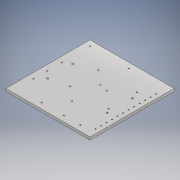
# Autodesk Inventor part: Base plate
Saved by Autodesk Inventor 2017 (Build 210142000, 142)
## iProperties
Created: 2016-09-16
Part Number: Base plate
Material: Aluminum 6061-AHC
Document SubType Name: Modeling
Designer: Andreas Fröderberg
Density: 2.7 g/cm^3
Appearance: Aluminum - Dark
Author: Andreas Fröderberg
Autodesk Inventor part; units mm, degrees
ref_plane "YZ Plane" through (0, 0, 0) normal (1, 0, 0) x (0, 1, 0)
ref_plane "XZ Plane" through (0, 0, 0) normal (0, 1, 0) x (-1, 0, 0)
ref_plane "XY Plane" through (0, 0, 0) normal (0, 0, 1) x (1, 0, 0)
sketch "Sketch1" plane through (0, 0, 0) normal (0, 0, 1) x (1, 0, 0)
  line L0 (0, 0) -> (305, 0)
  line L1 (305, 0) -> (305, 305)
  line L2 (305, 305) -> (0, 305)
  line L3 (0, 305) -> (0, 0)
  dimension "d0" = 305
  dimension "d1" = 305
  constraints: 8 end point, 2 parallel, 1 horizontal, 1 perpendicular
  measures "d0" distance of L2.end L1.end
  measures "d1" distance of L1.end L0.end
extrude "Extrusion1" add sketch "Sketch1" against normal blind 10
sketch "Sketch2" plane through (0, 0, 0) normal (0, 0, 1) x (1, 0, 0)
  line L0 (0, 305) -> (305, 305) projected
  line L1 (0, 305) -> (0, 0) projected
  point P0 (20, 285)
  point P1 (110, 225)
  dimension "d4" = 90
  dimension "d5" = 60
  dimension "d6" = 20
  dimension "d7" = 20
  measures "d4" horizontal distance of point (110, 225) point (20, 285)
  measures "d5" vertical distance of point (110, 225) point (20, 285)
  measures "d6" distance from line of L0 point (20, 285)
  measures "d7" distance from line of L1 point (20, 285)
hole "80x50" at (20, 285, 0) at (110, 225, 0) direction (0, 0, -1) diameter 4.134 depth 14.2 tip angle 118 thread size "M5x0.8" class "6H" standard "ISO Metric profile"
pattern_linear "Rectangular Pattern1" count 3 spacing 102.5 along (0, -1, 0) count 2 spacing 140 along (1, 0, 0) of "80x50"
sketch "Sketch4" plane through (0, 0, 0) normal (0, 0, 1) x (1, 0, 0)
  line L0 (0, 305) -> (0, 0) projected
  line L1 (305, 305) -> (0, 305) projected
  point P0 (290, 255)
  dimension "d40" = 290
  dimension "d41" = 50
  measures "d40" distance from line of L0 point (290, 255)
  measures "d41" distance from line of L1 point (290, 255)
hole "Magasin" at (290, 255, 0) direction (0, 0, -1) diameter 4.134 end through all thread size "M5x0.8" class "6H" standard "ISO Metric profile"
pattern_linear "Mag pat" count 12 spacing 20 along (0, -1, 0) of "Magasin"
sketch "Sketch5" plane through (0, 0, 0) normal (0, 0, 1) x (1, 0, 0)
  circle A0 centre (20, 285) radius 2.067 projected
  line L0 (0, 0) -> (305, 0) projected
  point P0 (190, 175)
  point P1 (20, 130)
  point P2 (190, 20)
  dimension "d42" = 170
  dimension "d43" = 110
  dimension "d44" = 20
  dimension "d45" = 110
  dimension "d46" = 170
  constraints: 1 vertical alignment
  measures "d42" horizontal distance of point (190, 175) A0.centre
  measures "d43" vertical distance of A0.centre point (190, 175)
  measures "d44" distance from line of L0 point (190, 20)
  measures "d45" vertical distance of point (190, 20) point (20, 130)
  measures "d46" horizontal distance of point (190, 20) point (20, 130)
hole "160x100" at (190, 175, 0) at (20, 130, 0) at (190, 20, 0) direction (0, 0, -1) diameter 4.134 depth 14.2 tip angle 118 thread size "M5x0.8" class "6H" standard "ISO Metric profile"
sketch "Fixture" plane through (0, 0, 0) normal (0, 0, 1) x (1, 0, 0)
  line L0 (0, 305) -> (0, 0) projected
  line L1 (305, 305) -> (0, 305) projected
  point P0 (44.5, 198)
  point P1 (260.5, 198)
  point P2 (260.5, 107)
  point P3 (44.5, 107)
  dimension "d54" = 216
  dimension "d55" = 91
  dimension "d56" = 44.5
  dimension "d57" = 107
  constraints: 2 horizontal alignment, 2 vertical alignment
  measures "d54" distance of point (260.5, 198) point (44.5, 198)
  measures "d55" distance of point (44.5, 107) point (44.5, 198)
  measures "d56" distance from line of L0 point (44.5, 198)
  measures "d57" distance from line of L1 point (44.5, 198)
hole "Hole4" at (44.5, 198, 0) at (260.5, 198, 0) at (260.5, 107, 0) at (44.5, 107, 0) direction (0, 0, -1) diameter 3.5 end through all counterbore diameter 6 counterbore depth 4
body "Solid1"
